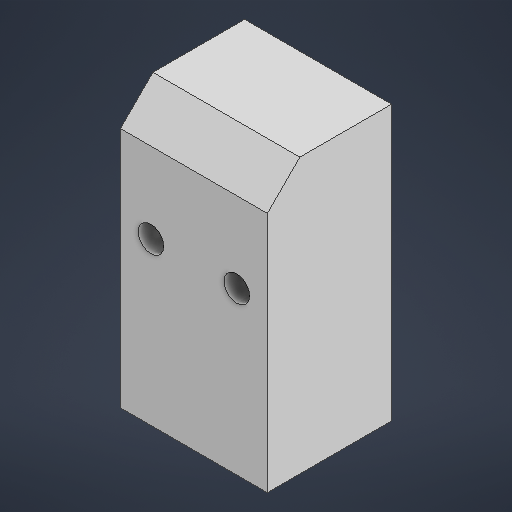
# Autodesk Inventor part: eddy
Saved by Autodesk Inventor 2025 (Build 290162000, 162)
## iProperties
Created: 2024-07-17
Part Number: eddy
Material: Generic
Document SubType Name: Modeling
Designer: Windows 7 was better
Density: 1 g/cm^3
Appearance: Default
Author: Windows 7 was better
Autodesk Inventor part; units mm, degrees
ref_plane "YZ Plane" through (0, 0, 0) normal (1, 0, 0) x (0, 1, 0)
ref_plane "XZ Plane" through (0, 0, 0) normal (0, 1, 0) x (-1, 0, 0)
ref_plane "XY Plane" through (0, 0, 0) normal (0, 0, 1) x (1, 0, 0)
sketch "Sketch1" plane through (0, 0, 0) normal (0, 0, 1) x (1, 0, 0)
  line L0 (0, 0) -> (18.1, 0)
  line L1 (18.1, 0) -> (18.1, 33.79)
  line L2 (18.1, 33.79) -> (0, 33.79)
  line L3 (0, 33.79) -> (0, 0)
  line L4 (0, 33.79) -> (0, 19.89) construction
  line L5 (0, 19.89) -> (18.1, 19.89) construction
  line L6 (9.05, 19.89) -> (14.34, 19.89) construction
  line L7 (14.34, 19.89) -> (3.76, 19.89) construction
  circle A0 centre (3.76, 19.89) radius 1.575
  circle A1 centre (14.34, 19.89) radius 1.575
  dimension "d0" = 18.1
  dimension "d1" = 33.79
  dimension "d2" = 13.9
  dimension "d3" = 5.29
  dimension "d4" = 10.58
  dimension "d5" = 3.15
  dimension "d6" = 3.15
  constraints: 16 end point, 4 point on line, 2 centre point, 2 coincident, 2 parallel, 2 perpendicular, 1 horizontal, 1 midpoint
  measures "d0" distance of L2.end L1.end
  measures "d1" distance of L1.end L0.end
  measures "d2" distance of L2.end L4.end
  measures "d3" distance of L6.start L6.end
  measures "d4" distance of L6.end L7.end
  measures "d5" diameter of A0
  measures "d6" diameter of A1
extrude "Extrusion1" add sketch "Sketch1" along normal blind 15.3
chamfer "Chamfer1" distance 4 angle 45 1 edges at (9.05, 33.79, 15.3)
body "Solid1"
